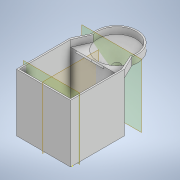
# Autodesk Inventor part: resoar
Saved by Autodesk Inventor 2021 (Build 250183000, 183)
## iProperties
Created: 2024-12-11
Part Number: resoar
Material: Generic
Document SubType Name: Modeling
Designer: 24oscnor
Density: 1 g/cm^3
Appearance: Default
Mass: 198.248 g
Surface Area: 1354.31 cm^2
Volume: 198.248 cm^3
Author: 24oscnor
Autodesk Inventor part; units mm, degrees
ref_plane "YZ Plane" through (0, 0, 0) normal (1, 0, 0) x (0, 1, 0)
ref_plane "XZ Plane" through (0, 0, 0) normal (0, 1, 0) x (-1, 0, 0)
ref_plane "XY Plane" through (0, 0, 0) normal (0, 0, 1) x (1, 0, 0)
sketch "Sketch2" plane through (0, 0, 0) normal (0, 1, 0) x (-1, 0, 0)
  line L0 (0, 0) -> (100, 0)
  line L1 (100, 0) -> (100, -100)
  line L2 (100, -100) -> (0, -100)
  line L3 (0, -100) -> (0, 0)
  dimension "d2" = 100
  dimension "d3" = 100
  constraints: 8 end point, 2 parallel, 1 horizontal, 1 perpendicular
  measures "d2" distance of L2.end L0.start
  measures "d3" distance of L0.start L0.end
extrude "Extrusion2" add sketch "Sketch2" along normal blind 3
sketch "Sketch3" plane through (0, 0, 0) normal (1, 0, 0) x (0, 0, -1)
  line L0 (0, 0) -> (100, 0)
  line L1 (100, 0) -> (100, 113)
  line L2 (100, 113) -> (0, 113)
  line L3 (0, 113) -> (0, 0)
  dimension "d6" = 100
  dimension "d7" = 113
  constraints: 8 end point, 2 parallel, 1 horizontal, 1 perpendicular
  measures "d6" distance of L0.start L0.end
  measures "d7" distance of L0.end L1.end
extrude "Extrusion3" add sketch "Sketch3" along normal blind 3
sketch "Sketch4" plane through (0, 3, 0) normal (0, 0, 1) x (1, 0, 0)
  line L0 (3, -3) -> (-100, -3) projected
  line L1 (3, -3) -> (-100, -3)
  line L2 (-100, -3) -> (-100, 110)
  line L3 (-100, 110) -> (3, 110)
  line L4 (3, 110) -> (3, -3)
  point P0 (0, -3)
  dimension "d10" = 113
  dimension "d11" = 103
  constraints: 8 end point, 2 parallel, 1 horizontal, 1 perpendicular
  measures "d10" distance of L1.end L2.end
  measures "d11" distance of L2.end L3.end
extrude "Extrusion4" add sketch "Sketch4" along normal blind 3
sketch "Sketch5" plane through (-100, 3, 0) normal (-1, 0, 0) x (0, 0, 1)
  line L0 (-100, -3) -> (3, -3) projected
  line L1 (-100, 110) -> (3, 110) projected
  line L2 (3, -3) -> (-100, -3)
  line L3 (-100, -3) -> (-100, 110)
  line L4 (-100, 110) -> (3, 110)
  line L5 (3, 110) -> (3, -3)
  point P0 (0, -3)
  point P1 (3, 110)
  constraints: 8 end point, 2 parallel, 1 horizontal, 1 perpendicular
extrude "Extrusion5" add sketch "Sketch5" along normal blind 3
sketch "Sketch6" plane through (0, 3, -100) normal (0, 0, -1) x (-1, 0, 0)
  line L0 (103, -3) -> (103, 110) projected
  line L1 (-3, -3) -> (103, -3)
  line L2 (103, -3) -> (103, 97)
  line L3 (103, 97) -> (-3, 97)
  line L4 (-3, 97) -> (-3, -3)
  point P0 (0, -3)
  dimension "d16" = 100
  constraints: 8 end point, 2 parallel, 1 horizontal, 1 perpendicular, 1 point on line
  measures "d16" distance of L3.end L1.start
extrude "Extrusion6" add sketch "Sketch6" along normal blind 3
sketch "Sketch7" plane through (3, 0, 0) normal (1, 0, 0) x (0, 0, -1)
  point P0 (0, 0)
ref_plane "Work Plane1" through (-50, 3, 0) normal (1, 0, 0) x (0, 0, -1)
sketch "Sketch8" plane through (-50, 3, 0) normal (1, 0, 0) x (0, 0, -1)
  line L0 (103, 97) -> (103, -3) projected
  line L1 (103, 97) -> (133.6418, 71.2885)
  line L2 (133.6418, 71.2885) -> (133.6418, 31.2885)
  line L3 (130.6418, 69.8896) -> (103, 93.0838)
  line L4 (133.6418, 31.2885) -> (130.6418, 51.2885)
  line L5 (130.6418, 51.2885) -> (130.6418, 69.8896)
  line L6 (103, 93.0838) -> (100, 95.6011)
  line L7 (100, 0) -> (100, 97) projected
  line L8 (100, 97) -> (103, 97) projected
  line L9 (103, 97) -> (103, 110)
  line L10 (100, 110) -> (100, 97) projected
  line L11 (103, 110) -> (100, 110)
  line L12 (100, 110) -> (100, 95.6011)
  line L13 (100, 95.6011) -> (100, 97)
  line L14 (140.6418, 31.2885) -> (140.6418, 72.7039) construction
  point P0 (0, -3)
  dimension "d20" = 40
  dimension "d21" = 50
  dimension "d22" = 40
  dimension "d24" = 3
  dimension "d27" = 20
  dimension "d28" = 18.6011
  dimension "d29" = 7
  constraints: 22 end point, 3 perpendicular, 3 vertical, 2 parallel, 2 point on line
  measures "d20" distance of L0.start L1.end
  measures "d21" angle of L1 L0
  measures "d22" distance of L1.end L2.end
  measures "d24" distance between parallel lines of L1 L3
  measures "d27" vertical distance of L2.end L4.end
  measures "d28" distance of L4.end L3.start
  measures "d29" distance between parallel lines of L2 L14
revolve "Revolution1" add sketch "Sketch8" angle 360 about axis through (-50, 34.2885, -140.6418) along (0, 1, 0)
ref_plane "Work Plane2" through (-50, 63.589, -130.6418) normal (0, 0, -1) x (-1, 0, 0)
sketch "Sketch9" plane through (-50, 63.589, -130.6418) normal (0, 0, -1) x (-1, 0, 0)
  line L0 (-15.3248, 36.411) -> (-53, 36.411) projected
  line L1 (-50, 49.411) -> (50, 49.411) projected
  line L2 (-40.4865, 36.411) -> (40.6129, 36.411)
  line L3 (40.6129, 36.411) -> (40.6129, 49.411)
  line L4 (40.6129, 49.411) -> (-40.4865, 49.411)
  line L5 (-40.4865, 49.411) -> (-40.4865, 36.411)
  point P0 (-50, -63.589)
  constraints: 8 end point, 2 parallel, 2 point on line, 1 horizontal, 1 perpendicular
extrude "Extrusion7" cut sketch "Sketch9" against normal up to surface (130.6418 mm away)
sketch "Sketch10" plane through (-100, 100, -100) normal (0, 1, 0) x (1, 0, 0)
  line L0 (89.3923, 30.6418) -> (86.2892, 30.6418) projected
  line L1 (103, 0) -> (103, 3) projected
  line L2 (89.3923, 30.6418) -> (103, 3)
  line L3 (-3, 3) -> (34.6752, 3) projected
  line L4 (103, 3) -> (-3, 3)
  line L5 (-3, 3) -> (10.6077, 30.6418)
  arc A0 (65.3248, 3) -> (34.6752, 3) centre (50, 40.6418) ccw projected
  point P0 (100, -100)
  constraints: 6 end point, 1 collinear, 1 point on circle
extrude "Extrusion8" add sketch "Sketch10" against normal blind 1.5 contours L2 L4 A0 | A0 L3 L5
sketch "Sketch11" plane through (-103, 100, -100) normal (0, 1, 0) x (1, 0, 0)
  line L0 (92.3923, 30.6418) -> (89.2892, 30.6418) projected
  line L1 (103, 0) -> (89.2892, 30.6418)
  arc A0 (68.3248, 3) -> (92.3923, 30.6418) centre (53, 40.6418) ccw projected
  line L2 (89.2892, 30.6418) -> (92.3923, 30.6418)
  line L3 (106, 3) -> (92.3923, 30.6418) projected
  line L4 (92.3923, 30.6418) -> (106, 3)
  line L5 (106, 0) -> (103, 0) projected
  line L6 (106, 3) -> (106, 0)
  line L7 (106, 0) -> (103, 0)
  line L8 (16.7108, 30.6418) -> (13.6077, 30.6418) projected
  line L9 (3, -100) -> (3, 0) projected
  line L10 (16.7108, 30.6418) -> (3, 0)
  line L11 (3, 0) -> (0, 0)
  line L12 (0, 0) -> (0, 3) projected
  line L13 (0, 0) -> (0, 3)
  line L14 (13.6077, 30.6418) -> (16.7108, 30.6418)
  line L15 (16.7108, 30.6418) -> (13.6077, 30.6418)
  line L16 (13.6077, 30.6418) -> (0, 3)
  point P0 (103, -100)
  dimension "d35" = 30.8097
  constraints: 22 end point, 4 collinear, 3 perpendicular, 1 horizontal
  measures "d35" distance of L14.start L12.end
extrude "Extrusion9" add sketch "Sketch11" along normal blind 13
ref_plane "Work Plane3" through (0, 3, -13) normal (0, 0, -1) x (-1, 0, 0)
sketch "Sketch13" plane through (-50, 3, 0) normal (1, 0, 0) x (0, 0, -1)
  line L0 (100, 0) -> (0, 0) projected
  line L1 (24, 0) -> (-2.4904, 18.5488)
  line L2 (-2.4904, 18.5488) -> (-0.7697, 21.0062)
  line L3 (-0.7697, 21.0062) -> (29.2303, 0)
  line L4 (12.4755, 11.7318) -> (125.6722, 173.3935)
  point P0 (0, -3)
  dimension "d39" = 35
  dimension "d41" = 3
  dimension "d42" = 30
  dimension "d44" = 24
  dimension "d54" = 90
  constraints: 8 end point, 3 point on line, 2 perpendicular
  measures "d39" angle of L0 L1
  measures "d41" distance of L1.end L2.end
  measures "d42" horizontal distance of L2.end L3.end
  measures "d44" distance of L0.end L1.start
  measures "d54" angle of L3 L4
extrude "Extrusion10" add sketch "Sketch13" along normal mid plane 30
sketch "Sketch14" plane through (-65, 20.5052, -4.2303) normal (0, 0.819152, -0.5735764) x (1, 0, 0)
  line L0 (0, 0) -> (30, 0) construction
  line L1 (15, 0) -> (15, 30.5194) construction
  line L2 (0, 30.5194) -> (30, 30.5194) construction
  circle A0 centre (15, 15.2597) radius 10.25
  point P0 (65, 8.296)
  dimension "d47" = 20.5
  constraints: 3 midpoint, 2 end point, 1 centre point
  measures "d47" diameter of A0
extrude "Extrusion11" cut sketch "Sketch14" against normal blind 3
sketch "Sketch21" plane through (-50, 3, 0) normal (1, 0, 0) x (0, 0, -1)
  line L0 (100, 97) -> (77.3726, 119.6274)
  line L1 (100, 97) -> (100, 0) projected
  line L2 (77.3726, 119.6274) -> (75.2513, 117.5061)
  line L3 (75.2513, 117.5061) -> (100, 92.7574)
  point P0 (0, -3)
  dimension "d55" = 45
  dimension "d56" = 3
  dimension "d57" = 35
  dimension "d59" = 90
  constraints: 6 end point, 1 parallel, 1 point on line
  measures "d55" angle of L1 L0
  measures "d56" distance between parallel lines of L0 L3
  measures "d57" distance of L2.end L3.end
  measures "d59" angle of L2 L0
extrude "Extrusion12" add sketch "Sketch21" along normal mid plane 30
equation "\"d3\" = d2"
equation "\"d16\" = d2"
body "Solid2"
